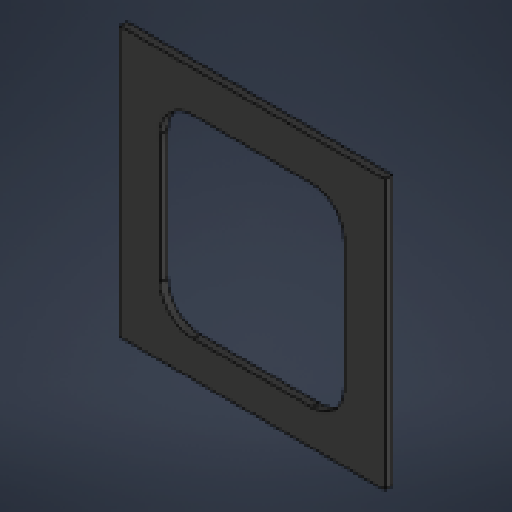
# Autodesk Inventor part: Door Panel Front Foam
Saved by Autodesk Inventor 2026 (Build 300175050, 175E)
## iProperties
Created: 2025-05-22
Part Number: Door Panel Front Foam
Material: Polyurethane Foam
Document SubType Name: Modeling
Designer: Joshua Eah
Density: 0.032 g/cm^3
Appearance: Coarse Textured - Umber
Mass: 5.58173 g
Surface Area: 647.191 cm^2
Volume: 174.429 cm^3
Author: Joshua Eah
Autodesk Inventor part; units mm, degrees
ref_plane "YZ Plane" through (0, 0, 0) normal (1, 0, 0) x (0, 1, 0)
ref_plane "XZ Plane" through (0, 0, 0) normal (0, 1, 0) x (-1, 0, 0)
ref_plane "XY Plane" through (0, 0, 0) normal (0, 0, 1) x (1, 0, 0)
sketch "Sketch1" plane through (0, 0, 0) normal (0, 0, 1) x (1, 0, 0)
  line L0 (0, 0) -> (230, 0)
  line L1 (230, 0) -> (230, 233.912)
  line L2 (230, 233.912) -> (0, 233.912)
  line L3 (0, 233.912) -> (0, 0)
  line L4 (38.1, 33.574) -> (191.9, 33.574)
  line L5 (191.9, 33.574) -> (191.9, 195.812)
  line L6 (191.9, 195.812) -> (38.1, 195.812)
  line L7 (38.1, 195.812) -> (38.1, 33.574)
  dimension "d0" = 230
  dimension "d1" = 233.912
  dimension "d2" = 33.574
  dimension "d3" = 38.1
  dimension "d4" = 38.1
  dimension "d5" = 38.1
  constraints: 16 end point, 4 parallel, 2 horizontal, 2 perpendicular
  measures "d0" distance of L2.end L1.end
  measures "d1" distance of L1.end L0.end
  measures "d2" distance between parallel lines of L0 L4
  measures "d3" distance between parallel lines of L3 L7
  measures "d4" distance between parallel lines of L1 L5
  measures "d5" distance between parallel lines of L2 L6
extrude "Extrusion1" add sketch "Sketch1" along normal blind 6.35
fillet "Fillet3" radius 25.4 4 edges at (191.9, 33.574, 3.175) (38.1, 33.574, 3.175) (38.1, 195.812, 3.175) (191.9, 195.812, 3.175)
thicken "Thicken2" operation cut thickness 3 both sides no extend neighbours yes toward (0, 1, 0) faces at (97.8333, 195.812, 4.2333) (38.1, 96.12, 2.1167) (191.9, 133.266, 4.2333) (132.1667, 33.574, 4.2333) (183.7764, 189.0315, 2.1167) (39.8558, 179.6917, 2.1167) (180.8083, 37.9875, 2.1167) (61.6019, 33.645, 2.1167)
equation "\"d4\" = d3"
body "Solid1"
